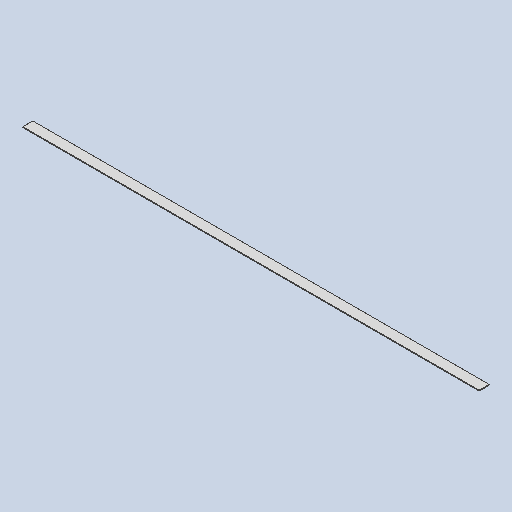
# Autodesk Inventor part: GBK bottom 0135
Saved by Autodesk Inventor 2026.2 (Build 302298000, 298)
## iProperties
Created: 2026-05-19
Part Number: GBK bottom 0135
Material: Steel
Document SubType Name: Sheet Metal
Designer: user
Density: 7.85 g/cm^3
Sheet Metal Rule: Default_mm
Appearance: Default
Mass: 7385.28 g
Surface Area: 4063.6 cm^2
Volume: 940.8 cm^3
Flat Pattern Width: 6.4 cm
Flat Pattern Length: 292 cm
Flat Pattern Area: 1868.8 cm^2
Sheet Metal Width: 64,000 mm
Sheet Metal Length: 2920,000 mm
Sheet Metal Area: 186880,000 mm^2
Stock Number: 0115
Engineer: 64
Author: user
Autodesk Inventor part; units mm, degrees
ref_plane "YZ Plane" through (0, 0, 0) normal (1, 0, 0) x (0, 1, 0)
ref_plane "XZ Plane" through (0, 0, 0) normal (0, 1, 0) x (-1, 0, 0)
ref_plane "XY Plane" through (0, 0, 0) normal (0, 0, 1) x (1, 0, 0)
sketch "Эскиз1" plane through (0, 0, 0) normal (0, 1, 0) x (-1, 0, 0)
  line L0 (1460, 32) -> (-1460, 32)
  line L1 (-1460, 32) -> (-1460, -32)
  line L2 (-1460, -32) -> (1460, -32)
  line L3 (1460, -32) -> (1460, 32)
  line L4 (1460, 32) -> (-1460, -32) construction
  line L5 (-1460, 32) -> (1460, -32) construction
  point P0 (0, 0)
  dimension "d0" = 2920
  dimension "d1" = 64
  measures "d0" distance of L2.end L1.end
  measures "d1" distance of L1.end L0.end
extrude "Пластина1" add sketch "Эскиз1" along normal blind 5
equation "\"d2\" = Толщина"
equation "\"Радиус_гибки\" = Толщина"
equation "\"Ширина_просечки\" = Толщина"
equation "\"Глубина_просечки\" = 0.5 * Толщина"
equation "\"Радиус_перехода\" = Радиус_гибки"
equation "\"Радиус_Якоби\" = Радиус_гибки"
equation "\"Размер_зазора\" = Толщина"
equation "\"Толщина\" = 5"
